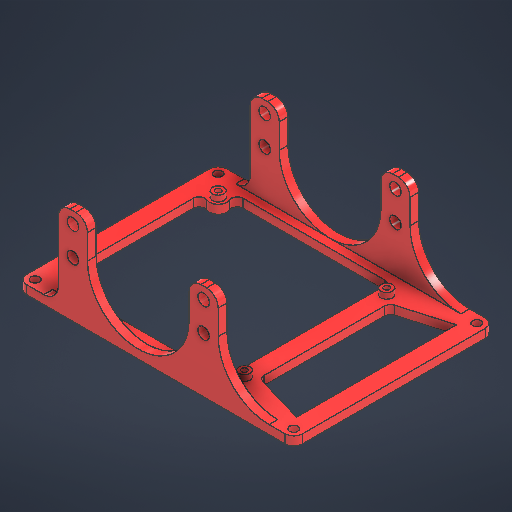
# Autodesk Inventor part: RP5_support
Saved by Autodesk Inventor 2026.1 (Build 301233000, 233)
## iProperties
Created: 2026-04-24
Part Number: RP5_support
Material: Generic
Document SubType Name: Modeling
Designer: emanuel
Density: 1 g/cm^3
Appearance: Default
Author: emanuel
Autodesk Inventor part; units mm, degrees
ref_plane "YZ Plane" through (0, 0, 0) normal (1, 0, 0) x (0, 1, 0)
ref_plane "XZ Plane" through (0, 0, 0) normal (0, 1, 0) x (-1, 0, 0)
ref_plane "XY Plane" through (0, 0, 0) normal (0, 0, 1) x (1, 0, 0)
sketch "Sketch1" plane through (0, 0, 0) normal (0, 1, 0) x (-1, 0, 0)
  line L0 (-29, -24.5) -> (29, -24.5)
  line L1 (29, -24.5) -> (29, 24.5)
  line L2 (29, 24.5) -> (-29, 24.5)
  line L3 (-29, 24.5) -> (-29, -24.5)
  line L4 (-29, -24.5) -> (29, 24.5) construction
  line L5 (29, -24.5) -> (-29, 24.5) construction
  circle A0 centre (29, 24.5) radius 1
  circle A1 centre (29, -24.5) radius 1
  circle A2 centre (-29, -24.5) radius 1
  circle A3 centre (-29, 24.5) radius 1
  circle A4 centre (29, 24.5) radius 2
  circle A5 centre (29, -24.5) radius 2
  circle A6 centre (-29, -24.5) radius 2
  circle A7 centre (-29, 24.5) radius 2
  line L6 (29, 24.5) -> (36, 24.5)
  line L7 (36, 24.5) -> (36, 31.5)
  line L8 (36, 31.5) -> (29, 31.5)
  line L9 (29, 31.5) -> (29, 24.5)
  circle A8 centre (36, 31.5) radius 1.5
  line L10 (-29, -24.5) -> (-53, -24.5)
  line L11 (-53, -24.5) -> (-53, -31.5)
  line L12 (-53, -31.5) -> (-29, -31.5)
  line L13 (-29, -31.5) -> (-29, -24.5)
  circle A9 centre (-53, -31.5) radius 1.5
  circle A10 centre (-53, -31.5) radius 3
  circle A11 centre (36, 31.5) radius 3
  line L14 (36, 31.5) -> (-53, 31.5)
  line L15 (-53, 31.5) -> (-53, -31.5)
  line L16 (-53, -31.5) -> (36, -31.5)
  line L17 (36, -31.5) -> (36, 31.5)
  circle A12 centre (36, -31.5) radius 1.5
  circle A13 centre (36, -31.5) radius 3
  circle A14 centre (-53, 31.5) radius 1.5
  circle A15 centre (-53, 31.5) radius 3
  line L18 (-53, 31.5) -> (-29, 24.5) construction
  line L19 (-52.16, 34.38) -> (-28.16, 27.38)
  line L20 (-29.84, 21.62) -> (-53.84, 28.62)
  arc A16 (-52.16, 34.38) -> (-53.84, 28.62) centre (-53, 31.5) ccw
  arc A17 (-29.84, 21.62) -> (-28.16, 27.38) centre (-29, 24.5) ccw
  line L21 (36, 31.5) -> (29, 24.5) construction
  line L22 (33.8787, 33.6213) -> (26.8787, 26.6213)
  line L23 (31.1213, 22.3787) -> (38.1213, 29.3787)
  arc A18 (38.1213, 29.3787) -> (33.8787, 33.6213) centre (36, 31.5) ccw
  arc A19 (26.8787, 26.6213) -> (31.1213, 22.3787) centre (29, 24.5) ccw
  line L24 (29, -24.5) -> (36, -31.5) construction
  line L25 (26.8787, -26.6213) -> (33.8787, -33.6213)
  line L26 (38.1213, -29.3787) -> (31.1213, -22.3787)
  arc A20 (31.1213, -22.3787) -> (26.8787, -26.6213) centre (29, -24.5) ccw
  arc A21 (33.8787, -33.6213) -> (38.1213, -29.3787) centre (36, -31.5) ccw
  line L27 (-53, -31.5) -> (-29, -24.5) construction
  line L28 (-52.16, -34.38) -> (-28.16, -27.38)
  line L29 (-29.84, -21.62) -> (-53.84, -28.62)
  arc A22 (-53.84, -28.62) -> (-52.16, -34.38) centre (-53, -31.5) ccw
  arc A23 (-28.16, -27.38) -> (-29.84, -21.62) centre (-29, -24.5) ccw
  point P0 (0, 0)
  point P1 (-41, 28)
  point P2 (32.5, 28)
  point P3 (32.5, -28)
  point P4 (-41, -28)
  dimension "d0" = 58
  dimension "d1" = 49
  dimension "d2" = 2
  dimension "d3" = 2
  dimension "d4" = 2
  dimension "d5" = 2
  dimension "d6" = 4
  dimension "d7" = 4
  dimension "d8" = 4
  dimension "d9" = 4
  dimension "d11" = 7
  dimension "d12" = 7
  dimension "d13" = 3
  dimension "d14" = 24
  dimension "d15" = 7
  dimension "d16" = 3
  dimension "d17" = 6
  dimension "d18" = 6
  dimension "d19" = 3
  dimension "d20" = 6
  dimension "d21" = 3
  dimension "d22" = 6
  dimension "d28" = 6
  constraints: 68 end point, 24 centre point, 16 coincident, 16 point on circle, 16 tangent, 12 parallel, 6 midpoint, 4 horizontal, 4 perpendicular, 3 concentric
  measures "d0" distance of L2.end L1.end
  measures "d1" distance of L1.end L0.end
  measures "d2" diameter of A0
  measures "d3" diameter of A1
  measures "d4" diameter of A2
  measures "d5" diameter of A3
  measures "d6" diameter of A4
  measures "d7" diameter of A5
  measures "d8" diameter of A6
  measures "d9" diameter of A7
  measures "d11" distance of L8.end L7.end
  measures "d12" distance of L7.end L6.end
  measures "d13" diameter of A8
  measures "d14" distance of L12.end L11.end
  measures "d15" distance of L11.end L10.end
  measures "d16" diameter of A9
  measures "d17" diameter of A10
  measures "d18" diameter of A11
  measures "d19" diameter of A12
  measures "d20" diameter of A13
  measures "d21" diameter of A14
  measures "d22" diameter of A15
  measures "d28" distance between parallel lines of L19 L20
extrude "Extrusion1" add sketch "Sketch1" along normal blind 3 contours A2 L3 A6 L0 | L0 A6 L13 A2 | A2 L10 A6 L3 | A2 L13 A6 L10 | A6 L3 A23 L0 | L0 A23 L28 L13 A6 | A6 L10 L29 A23 L3 | A6 L13 L28 L12 A10 L11 L29 L10 | A20 L1 A5 L0 | L0 A5 L1 A20 L26 L17 A13 L16 L25 | A17 L20 L15 A15 L14 L19 L2 A7 L3 | L3 A7 L2 A17 | L11 A10 L29 | L28 A10 L12 | A5 L1 A1 L0 | L0 A1 L1 A5 | A7 L2 A3 L3 | L3 A3 L2 A7 | L20 A15 L15 | A10 L12 A9 L11 | L11 A9 L12 A10 | L16 A13 L25 | A19 L2 A4 L1 | L1 A4 L6 L23 A19 | A19 L22 L9 A4 L2 | A15 L14 A14 L15 | L15 A14 L14 A15 | A13 L17 A12 L16 | L16 A12 L17 A13 | A4 L2 A0 L1 | L1 A0 L6 A4 | L26 A13 L17 | A4 L9 A0 L2 | L14 A15 L19 | L6 A0 L9 A4 | A4 L9 L22 L8 A11 L7 L23 L6 | L7 A11 L23 | L22 A11 L8 | A11 L8 A8 L7 | L7 A8 L8 A11
extrude "Extrusion2" add sketch "Sketch1" along normal blind 5 contours A2 L3 A6 L0 | L0 A6 L13 A2 | A2 L10 A6 L3 | A2 L13 A6 L10 | A5 L1 A1 L0 | L0 A1 L1 A5 | A7 L2 A3 L3 | L3 A3 L2 A7 | A4 L2 A0 L1 | L1 A0 L6 A4 | A4 L9 A0 L2 | L6 A0 L9 A4
sketch "Sketch2" plane through (0, 3, 0) normal (0, 1, 0) x (1, 0, 0)
  circle A0 centre (29, 24.5) radius 1 projected
  circle A1 centre (-29, -24.5) radius 1 projected
  line L0 (29, 24.5) -> (-29, 24.5)
  line L1 (-29, 24.5) -> (-29, -24.5)
  line L2 (-29, -24.5) -> (29, -24.5)
  line L3 (29, -24.5) -> (29, 24.5)
  circle A2 centre (53, 31.5) radius 1.5 projected
  circle A3 centre (-36, -31.5) radius 1.5 projected
  line L4 (53, 31.5) -> (-36, 31.5)
  line L5 (-36, 31.5) -> (-36, -31.5)
  line L6 (-36, -31.5) -> (53, -31.5)
  line L7 (53, -31.5) -> (53, 31.5)
  line L8 (-36, 31.5) -> (-36, -31.5) construction
  line L9 (-33, 31.5) -> (-33, -31.5)
  line L10 (-39, -31.5) -> (-39, 31.5)
  arc A4 (-33, 31.5) -> (-39, 31.5) centre (-36, 31.5) ccw
  arc A5 (-39, -31.5) -> (-33, -31.5) centre (-36, -31.5) ccw
  line L11 (-36, -31.5) -> (53, -31.5) construction
  line L12 (-36, -28.5) -> (53, -28.5)
  line L13 (53, -34.5) -> (-36, -34.5)
  arc A6 (-36, -28.5) -> (-36, -34.5) centre (-36, -31.5) ccw
  arc A7 (53, -34.5) -> (53, -28.5) centre (53, -31.5) ccw
  circle A8 centre (53, -31.5) radius 1.5 projected
  line L14 (53, -31.5) -> (53, 31.5) construction
  line L15 (50, -31.5) -> (50, 31.5)
  line L16 (56, 31.5) -> (56, -31.5)
  arc A9 (50, -31.5) -> (56, -31.5) centre (53, -31.5) ccw
  arc A10 (56, 31.5) -> (50, 31.5) centre (53, 31.5) ccw
  line L17 (53, 31.5) -> (-36, 31.5) construction
  line L18 (53, 28.5) -> (-36, 28.5)
  line L19 (-36, 34.5) -> (53, 34.5)
  arc A11 (53, 28.5) -> (53, 34.5) centre (53, 31.5) ccw
  arc A12 (-36, 34.5) -> (-36, 28.5) centre (-36, 31.5) ccw
  line L20 (29, 24.5) -> (29, -24.5) construction
  line L21 (26, 24.5) -> (26, -24.5)
  line L22 (32, -24.5) -> (32, 24.5)
  arc A13 (32, 24.5) -> (26, 24.5) centre (29, 24.5) ccw
  arc A14 (26, -24.5) -> (32, -24.5) centre (29, -24.5) ccw
  circle A15 centre (-36, 31.5) radius 1.5
  circle A16 centre (-36, -31.5) radius 1.5
  circle A17 centre (53, -31.5) radius 1.5
  circle A18 centre (53, 31.5) radius 1.5
  circle A19 centre (29, 24.5) radius 1
  circle A20 centre (29, -24.5) radius 1
  point P0 (0, 0)
  point P1 (-36, 0)
  point P2 (8.5, -31.5)
  point P3 (53, 0)
  point P4 (8.5, 31.5)
  point P5 (29, 0)
  point P6 (50, 28.5)
  point P7 (50, -28.5)
  point P8 (-33, -28.5)
  point P9 (-33, 28.5)
  dimension "d27" = 6
  constraints: 56 end point, 20 point on circle, 20 tangent, 16 centre point, 11 equal length, 6 coincident, 5 midpoint, 5 perpendicular, 3 concentric, 2 horizontal
  measures "d27" diameter of A14
extrude "Extrusion3" add sketch "Sketch2" against normal blind 3 contours A0 L0 A13 L22 A14 L2 A20 L3 | A0 L3 A20 L2 L21 L0 | L15 L18 L9 L4 | L4 A4 L19 A10 | A11 L16 A7 L7 | L7 L12 L15 L18 | L9 L18 L5 A15 L4 | L4 A15 L5 A12 A4 | A7 A9 L6 A8 L7 | L7 A8 L6 L15 L12 | L9 L12 L5 L18 | L15 L6 L9 L12 | L9 L6 A3 L5 L12 | L5 A6 L10 A12 | A9 L13 A5 L6 | A5 A6 L5 A3 L6
fillet "Fillet1" radius 2 8 edges at (-28.7574, 1.5, 28.5) (-33, 1.5, 24.2574) (32, 1.5, -22.25) (32, 1.5, 22.25) (32, 1.5, 28.5) (32, 1.5, -28.5) (-28.7574, 1.5, -28.5) (-33, 1.5, -24.2574)
sketch "Sketch3" plane through (0, 3, 0) normal (0, 1, 0) x (1, 0, 0)
  line L0 (-36, 34.5) -> (53, 34.5) projected
  line L1 (53, -34.5) -> (-36, -34.5) projected
  line L2 (0, 34.5) -> (20, 34.5)
  line L3 (20, 34.5) -> (20, -34.5)
  line L4 (20, -34.5) -> (0, -34.5)
  line L5 (0, -34.5) -> (0, 34.5)
  line L6 (0, 34.5) -> (-15, 34.5)
  line L7 (-15, 34.5) -> (-15, -34.5)
  line L8 (-15, -34.5) -> (0, -34.5)
  line L9 (0, -34.5) -> (0, 34.5)
  line L10 (-15, 34.5) -> (-25, 34.5)
  line L11 (-25, 34.5) -> (-25, 31.5)
  line L12 (-25, 31.5) -> (-15, 31.5)
  line L13 (-15, 31.5) -> (-15, 34.5)
  line L14 (20, 34.5) -> (30, 34.5)
  line L15 (30, 34.5) -> (30, 31.5)
  line L16 (30, 31.5) -> (20, 31.5)
  line L17 (20, 31.5) -> (20, 34.5)
  line L18 (-15, -34.5) -> (-25, -34.5)
  line L19 (-25, -34.5) -> (-25, -31.5)
  line L20 (-25, -31.5) -> (-15, -31.5)
  line L21 (-15, -31.5) -> (-15, -34.5)
  line L22 (20, -34.5) -> (30, -34.5)
  line L23 (30, -34.5) -> (30, -31.5)
  line L24 (30, -31.5) -> (20, -31.5)
  line L25 (20, -31.5) -> (20, -34.5)
  point P0 (0, 0)
  dimension "d32" = 20
  dimension "d33" = 15
  dimension "d34" = 10
  dimension "d35" = 3
  dimension "d36" = 10
  dimension "d37" = 3
  dimension "d38" = 10
  dimension "d39" = 3
  dimension "d40" = 10
  dimension "d41" = 3
  constraints: 48 end point, 12 parallel, 6 horizontal, 6 perpendicular, 3 point on line
  measures "d32" distance of L3.end L4.end
  measures "d33" distance of L8.end L7.end
  measures "d34" distance of L12.end L11.end
  measures "d35" distance of L11.end L10.end
  measures "d36" distance of L15.end L16.end
  measures "d37" distance of L14.end L15.end
  measures "d38" distance of L19.end L20.end
  measures "d39" distance of L18.end L19.end
  measures "d40" distance of L24.end L23.end
  measures "d41" distance of L23.end L22.end
extrude "Extrusion4" add sketch "Sketch3" along normal blind 30 contours L0 L7 L12 L11 | L0 L15 L16 L3 | L7 L1 L19 L20 | L3 L24 L23 L1
fillet "Fillet2" radius 17.5 4 edges at (-15, 3, 33) (20, 3, 33) (-15, 3, -33) (20, 3, -33)
fillet "Fillet3" radius 17.5 2 edges at (30, 3, -33) (30, 3, 33)
fillet "Fillet4" radius 5 2 edges at (-25, 3, 33) (-25, 3, -33)
sketch "Sketch4" plane through (-36, 0, 34.5) normal (0, 0, 1) x (1, 0, 0)
  line L0 (11, 8) -> (11, 33) projected
  line L1 (11, 33) -> (16, 33)
  line L2 (16, 33) -> (16, 29)
  line L3 (16, 29) -> (11, 29)
  line L4 (11, 29) -> (11, 33)
  line L5 (66, 20.5) -> (66, 33) projected
  line L6 (66, 33) -> (61, 33)
  line L7 (61, 33) -> (61, 29)
  line L8 (61, 29) -> (66, 29)
  line L9 (66, 29) -> (66, 33)
  circle A0 centre (61, 29) radius 2
  circle A1 centre (16, 29) radius 2
  point P0 (36, 0)
  dimension "d47" = 5
  dimension "d48" = 4
  dimension "d49" = 5
  dimension "d50" = 4
  dimension "d51" = 4
  dimension "d52" = 4
  constraints: 16 end point, 4 parallel, 2 centre point, 2 coincident, 2 horizontal, 2 perpendicular
  measures "d47" distance of L2.end L3.end
  measures "d48" distance of L1.end L2.end
  measures "d49" distance of L8.end L7.end
  measures "d50" distance of L7.end L6.end
  measures "d51" diameter of A0
  measures "d52" diameter of A1
extrude "Extrusion5" cut sketch "Sketch4" against normal up to surface (69 mm away) contours A1 L2 L3 | L3 L2 A1 | A0 L7 L8 | L8 L7 A0
fillet "Fillet5" radius 4 8 edges at (30, 33, 33) (20, 33, 33) (-15, 33, 33) (-25, 33, 33) (30, 33, -33) (20, 33, -33) (-15, 33, -33) (-25, 33, -33)
sketch "Sketch5" plane through (-36, 0, 34.5) normal (0, 0, 1) x (1, 0, 0)
  circle A0 centre (16, 29) radius 2 projected
  line L0 (16, 29) -> (61, 29)
  line L1 (61, 29) -> (61, 19)
  line L2 (61, 19) -> (16, 19)
  line L3 (16, 19) -> (16, 29)
  circle A1 centre (16, 19) radius 2
  circle A2 centre (61, 19) radius 2
  point P0 (36, 0)
  dimension "d56" = 10
  dimension "d57" = 4
  dimension "d58" = 4
  constraints: 8 end point, 2 centre point, 2 coincident, 2 parallel, 1 horizontal, 1 perpendicular
  measures "d56" distance of L0.end L1.end
  measures "d57" diameter of A1
  measures "d58" diameter of A2
extrude "Extrusion6" cut sketch "Sketch5" against normal up to surface (69 mm away) contours A1 L2 L3 | L3 L2 A1 | A2 L2 L1 | L1 L2 A2
body "Solid1"
